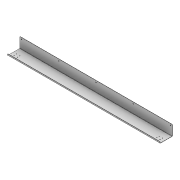
# Autodesk Inventor part: DragChain_Guide_A
Saved by Autodesk Inventor 2020 (Build 240168000, 168)
## iProperties
Created: 2021-12-05
Part Number: DragChain_Guide_A
Material: 一般
Document SubType Name: Sheet Metal
Designer: ken113
Density: 1 g/cm^3
Sheet Metal Rule: Default_mm
Appearance: 既定
Author: ken113
Autodesk Inventor part; units mm, degrees
ref_plane "YZ Plane" through (0, 0, 0) normal (1, 0, 0) x (0, 1, 0)
ref_plane "XZ Plane" through (0, 0, 0) normal (0, 1, 0) x (-1, 0, 0)
ref_plane "XY Plane" through (0, 0, 0) normal (0, 0, 1) x (1, 0, 0)
sketch "スケッチ1" plane through (0, 0, 0) normal (0, 0, 1) x (1, 0, 0)
  line L0 (475, -31) -> (-475, -31)
  line L1 (-475, -31) -> (-475, 31)
  line L2 (-475, 31) -> (475, 31)
  line L3 (475, 31) -> (475, -31)
  line L4 (475, -31) -> (-475, 31) construction
  line L5 (-475, -31) -> (475, 31) construction
  point P0 (0, 0)
  dimension "d0" = 62
  dimension "d1" = 950
  measures "d0" distance of L0.end L1.end
  measures "d1" distance of L1.end L2.end
extrude "プレート1" add sketch "スケッチ1" along normal blind 1.5
sketch "スケッチ2" plane through (475, -32.5, 3) normal (0, -1, 0) x (1, 0, 0)
  line L0 (-950, 0) -> (0, 0)
  line L1 (0, 0) -> (0, 72)
  line L2 (0, 72) -> (-950, 72)
  line L3 (-950, 72) -> (-950, 0)
  constraints: 6 end point, 1 horizontal, 1 perpendicular, 1 vertical
edge flange "フランジ1" height 75 angle 90 thickness 1.5 bend radius 1.5 thickness toward (0, -1, 0) relief straight relief width 1.5 relief depth 0.75 edges at (0, -31, 1.5) wall of the first edge with corners at (-475, -32.5, 3) (475, -32.5, 3) (475, -32.5, 75) (-475, -32.5, 75)
bend "曲げ1"
corner "コーナー1"
sketch "スケッチ3" plane through (475, -31, 76.5) normal (0, 0, 1) x (1, 0, 0)
  line L0 (-950, 0) -> (0, 0)
  line L1 (0, 0) -> (0, 7)
  line L2 (0, 7) -> (-950, 7)
  line L3 (-950, 7) -> (-950, 0)
  constraints: 6 end point, 1 horizontal, 1 perpendicular, 1 vertical
edge flange "フランジ2" height 10 angle 90 thickness 1.5 bend radius 1.5 thickness toward (0, 0, 1) relief straight relief width 1.5 relief depth 0.75 edges at (0, -32.5, 75) wall of the first edge with corners at (-475, -31, 76.5) (475, -31, 76.5) (475, -24, 76.5) (-475, -24, 76.5)
bend "曲げ2"
corner "コーナー2"
sketch "スケッチ4" plane through (0, 0, 1.5) normal (0, 0, 1) x (1, 0, 0)
  line L0 (-475, -31) -> (-475, 31) projected
  line L1 (475, -31) -> (-475, -31) projected
  line L2 (475, 31) -> (475, -31) projected
  line L3 (-475, 31) -> (475, 31) projected
  line L4 (-465, 21) -> (465, 21)
  point P0 (0, 0)
  point P1 (-232.5, 21)
  point P2 (0, 21)
  point P3 (232.5, 21)
  dimension "d23" = 10
  dimension "d24" = 10
  dimension "d25" = 10
  dimension "d26" = 930
  dimension "d27" = 232.5
  dimension "d28" = 232.5
  dimension "d29" = 232.5
  constraints: 2 end point, 2 point on line, 1 coincident, 1 horizontal, 1 midpoint
  measures "d23" distance between parallel lines of L3 L4
  measures "d24" distance from line of L4.start L0
  measures "d25" distance from line of L2 L4.end
  measures "d26" distance of L4.start L4.end
  measures "d27" distance of point (-232.5, 21) point (-465, 21)
  measures "d28" distance of point (0, 21) point (-232.5, 21)
  measures "d29" distance of point (232.5, 21) point (0, 21)
hole "穴1" at (-465, 21, 1.5) at (-232.5, 21, 1.5) at (0, 21, 1.5) at (232.5, 21, 1.5) at (465, 21, 1.5) direction (0, 0, -1) diameter 5.3 end through all
sketch "スケッチ5" plane through (-475, -32.5, 3) normal (0, 1, 0) x (1, 0, 0)
  line L0 (950, 0) -> (0, 0) projected
  line L1 (0, -72) -> (0, 0) projected
  line L2 (0, -72) -> (950, -72) projected
  line L3 (950, -72) -> (950, 0) projected
  line L4 (930, -54) -> (930, -39)
  line L5 (0, 1.5) -> (950, 1.5) projected
  line L6 (930, -54) -> (910, -54)
  line L7 (910, -54) -> (910, -39)
  line L8 (910, -39) -> (930, -39)
  line L9 (930, -39) -> (930, -54)
  point P0 (475, 3)
  point P1 (930, -46.5)
  dimension "d37" = 15
  dimension "d38" = 48
  dimension "d39" = 20
  dimension "d40" = 20
  constraints: 10 end point, 2 parallel, 1 horizontal, 1 horizontal alignment, 1 midpoint, 1 perpendicular, 1 vertical
  measures "d37" distance of L4.end L4.start
  measures "d38" distance from line of point (930, -46.5) L5
  measures "d39" distance from line of L3 L4.end
  measures "d40" distance of L4.start L6.end
hole "穴2" at (455, -32.5, 57) at (455, -32.5, 42) at (435, -32.5, 57) at (435, -32.5, 42) direction (0, -1, 0) diameter 3.242 end through all thread size "M4x0.7" class "6H" standard "ISO Metric profile"
mirror "ミラー1" about plane through (0, 0, 0) normal (1, 0, 0) of "穴2"
fillet "フィレット1" radius 2 4 edges at (-475, -24, 77.25) (-475, 31, 0.75) (475, -24, 77.25) (475, 31, 0.75)
equation "\"d27\" = 0.25 * d26"
equation "\"d28\" = d27"
equation "\"d29\" = d27"
equation "\"d35\" = Thickness"
equation "\"d2\" = Thickness"
equation "\"d3\" = BendReliefWidth"
equation "\"d4\" = BendReliefDepth"
equation "\"d5\" = MinimumRemnant"
equation "\"d6\" = TransitionRadius"
equation "\"d9\" = BendRadius"
equation "\"d10\" = CornerReliefSize"
equation "\"d11\" = GapSize"
equation "\"d12\" = JacobiRadiusSize"
equation "\"d13\" = BendReliefWidth"
equation "\"d14\" = BendReliefDepth"
equation "\"d15\" = MinimumRemnant"
equation "\"d16\" = TransitionRadius"
equation "\"d19\" = BendRadius"
equation "\"d20\" = CornerReliefSize"
equation "\"d21\" = GapSize"
equation "\"d22\" = JacobiRadiusSize"
equation "\"BendRadius\" = Thickness"
equation "\"BendReliefWidth\" = Thickness"
equation "\"BendReliefDepth\" = 0.5 * Thickness"
equation "\"CornerReliefSize\" = 4 * Thickness"
equation "\"MinimumRemnant\" = 2 * Thickness"
equation "\"TransitionRadius\" = BendRadius"
equation "\"JacobiRadiusSize\" = BendRadius"
equation "\"GapSize\" = Thickness"
equation "\"Thickness\" = 1.5"
